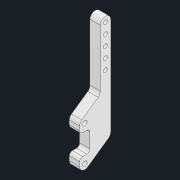
# Autodesk Inventor part: shooter_base8[
Saved by Autodesk Inventor 2022 (Build 260153000, 153)
## iProperties
Created: 2021-11-15
Part Number: shooter_base8[
Material: ABS プラスチック
Document SubType Name: Modeling
Designer: Yuta Kage
Density: 1.06 g/cm^3
Appearance: 滑らか - 白
Author: Yuta Kage
Autodesk Inventor part; units mm, degrees
ref_plane "YZ Plane" through (0, 0, 0) normal (1, 0, 0) x (0, 1, 0)
ref_plane "XZ Plane" through (0, 0, 0) normal (0, 1, 0) x (-1, 0, 0)
ref_plane "XY Plane" through (0, 0, 0) normal (0, 0, 1) x (1, 0, 0)
sketch "スケッチ1" plane through (0, 0, 0) normal (1, 0, 0) x (0, 1, 0)
  line L0 (0, 0) -> (21.0062, -30)
  line L1 (21.0062, -30) -> (123, -30)
  line L2 (123, -30) -> (123, -20)
  line L3 (123, -20) -> (60.2119, -20)
  line L4 (60.2119, -20) -> (46.2077, 0)
  line L5 (46.2077, 0) -> (0, 0)
  line L6 (0, 6) -> (0, -36) projected
  point P0 (9.6049, -5)
  point P1 (43.6049, -5)
  dimension "d1" = 35
  dimension "d2" = 10
  dimension "d3" = 123
  dimension "d4" = 30
  dimension "d19" = 5
  dimension "d20" = 5
  dimension "d21" = 5
  dimension "d22" = 5
  dimension "d23" = 34
  constraints: 12 end point, 2 parallel, 2 perpendicular, 1 horizontal
  measures "d1" angle of L0 L6
  measures "d2" distance of L1.end L2.end
  measures "d3" distance between parallel lines of L2 L6
  measures "d4" distance between parallel lines of L5 L1
  measures "d19" distance from line of L5 point (9.605, -5)
  measures "d20" distance from line of point (9.605, -5) L0
  measures "d21" distance from line of L5 point (43.605, -5)
  measures "d22" distance from line of L4 point (43.605, -5)
  measures "d23" distance of point (9.605, -5) point (43.605, -5)
extrude "押し出し1" add sketch "スケッチ1" along normal mid plane 10
sketch "スケッチ2" plane through (5, 0, 0) normal (1, 0, 0) x (0, 0, -1)
  line L0 (0, 46.2077) -> (0, 0) projected
  line L1 (0, 0) -> (30, 21.0062) projected
  point P0 (5, 43.6049)
  point P1 (5, 9.6049)
  dimension "d9" = 5
  dimension "d10" = 5
  dimension "d11" = 34
  constraints: 1 vertical alignment
  measures "d9" distance from line of L0 point (5, 9.605)
  measures "d10" distance from line of L1 point (5, 9.605)
  measures "d11" distance of point (5, 43.605) point (5, 9.605)
hole "穴1" at (5, 43.6049, -5) at (5, 9.6049, -5) direction (-1, 0, 0) diameter 4.5 end through all clearance for "Flat Head Machine Screw" size "M4" standard "Ansi Metric M Profile"
fillet "フィレット1" radius 5 4 edges at (0, 60.2119, -20) (0, 46.2077, 0) (0, 0, 0) (0, 21.0062, -30)
fillet "フィレット2" radius 5 2 edges at (0, 123, -20) (0, 123, -30)
sketch "スケッチ3" plane through (5, 0, 0) normal (1, 0, 0) x (0, 0, -1)
  arc A0 (30, 118) -> (20, 118) centre (25, 118) ccw projected
  point P0 (0, 0)
hole "穴2" at (5, 118, -25) direction (-1, 0, 0) diameter 4 end through all
pattern_linear "矩形状パターン1" count 5 spacing 10 along (0, -1, 0) of "穴2"
sketch "スケッチ4" plane through (-5, 0, 0) normal (-1, 0, 0) x (0, 0, 1)
  line L0 (0, 36.6049) -> (-10, 36.6049)
  line L1 (-10, 36.6049) -> (-10, 16.6049)
  line L2 (-10, 16.6049) -> (0, 16.6049)
  line L3 (0, 16.6049) -> (0, 36.6049)
  line L4 (0, 9.6049) -> (0, 43.6049) projected
  circle A0 centre (-5, 43.6049) radius 2.25 projected
  circle A1 centre (-5, 9.6049) radius 2.25 projected
  point P0 (0, 0)
  dimension "d38" = 10
  dimension "d39" = 7
  dimension "d40" = 7
  constraints: 8 end point, 2 parallel, 1 horizontal, 1 perpendicular, 1 point on line
  measures "d38" distance between parallel lines of L4 L1
  measures "d39" distance from line of L0 A0.centre
  measures "d40" distance from line of A1.centre L2
extrude "押し出し2" cut sketch "スケッチ4" against normal through all contours L3 L2 L1 L0
fillet "フィレット3" radius 3 4 edges at (0, 36.6049, 0) (0, 36.6049, -10) (0, 16.6049, -10) (0, 16.6049, 0)
